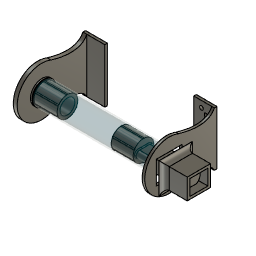
door-window-v3 (Autodesk Fusion 360 design; units mm, degrees)
Autodesk Fusion 360 part; units mm, degrees
note: some values were not read from the file. Chosen so that the rebuilt part matches the saved one: which face or edge a step refers to. Set by a fixed rule: which sketch regions a step uses.
sketch "left holder" plane through (0, 0, 0) normal (1, 0, 0) x (0, 1, 0)
  circle A0 centre (0, 0) radius 8
  circle A1 centre (0, 0) radius 9
  line L0 (0, 0) -> (36, 0) construction
  line L1 (35, 21) -> (37, 21)
  line L2 (37, 21) -> (37, -21)
  line L3 (37, -21) -> (35, -21)
  line L4 (35, -21) -> (35, 21)
  line L5 (35, 21) -> (37, -21) construction
  line L6 (37, 21) -> (35, -21) construction
  circle A2 centre (0, 0) radius 19
  spline S0 degree 5 poles (7.0865, 17.629) (9.067, 17.0403) (12.8106, 16.0316) (17.775, 15.0239) (23.2427, 14.5868) (28.5965, 15.294) (31.8536, 16.8398) (33.6847, 18.6426) (34.6107, 20.1614) (35, 21) knots 0 0 0 0 0 0 0.2 0.4 0.6 0.8 1 1 1 1 1 1
  line L7 (2.4318, 19.0126) -> (11.7413, 16.2454)
  line L8 (34.2297, 19.3403) -> (35.7703, 22.6597)
  spline S1 degree 5 poles (7.0865, -17.629) (9.067, -17.0403) (12.8106, -16.0316) (17.775, -15.0239) (23.2427, -14.5868) (28.5965, -15.294) (31.8536, -16.8398) (33.6847, -18.6426) (34.6107, -20.1614) (35, -21) knots 0 0 0 0 0 0 0.2 0.4 0.6 0.8 1 1 1 1 1 1
  line L9 (2.4318, -19.0126) -> (11.7413, -16.2454)
  line L10 (34.2297, -19.3403) -> (35.7703, -22.6597)
  circle A3 centre (0, 0) radius 3
  point P0 (36, 0)
  dimension "d1" = 16
  dimension "d2" = 18
  dimension "d3" = 36
  dimension "d4" = 2
  dimension "d5" = 42
  dimension "d8" = 38
  dimension "d9" = 6
  constraint coincident A0.centre A1.centre
  constraint concentric A0 A1
  constraint horizontal L0
  constraint horizontal L1
  constraint perpendicular L1 L2
  constraint parallel L1 L3
  constraint parallel L2 L4
  constraint coincident L5 P0
  constraint coincident L6 P0
  constraint coincident P0 L0.end
  constraint concentric A1 A2
  constraint coincident A2 S0.start
  constraint midpoint S0.start L7
  constraint midpoint L1.start L8
  constraint symmetric L0 L1.start L3.end
  constraint symmetric L0 S0.start S1.start
  constraint symmetric L0 L7.start L9.start
  constraint symmetric L0 L7.end L9.end
  constraint symmetric L0 L8.start L10.start
  constraint symmetric L0 L8.end L10.end
  measures "d1" diameter of A0
  measures "d2" diameter of A1
  measures "d3" distance of A0.centre P0
  measures "d4" distance of L2.end L3.end
  measures "d5" distance of L1.end L2.end
  measures "d8" diameter of A2
  measures "d9" diameter of A3
extrude "Extrude1" add sketch "left holder" along normal blind 17 contours L1 L2 L3 L4 makes body 1
extrude "Extrude3" add sketch "left holder" along normal blind 2 contours A0 | A1 | L4 A2 S0 S1 | A2 L7 | A2 L7 L9 | A2 L9 bodies 1
extrude "Extrude4" add sketch "left holder" along normal blind 90 from surface at 5 separate body contours A1 makes body 2
extrude "Extrude5" add sketch "left holder" along normal blind 10 from surface at 3 separate body contours A0 | A3 makes body 3
extrude "Extrude6" add sketch "left holder" against normal blind 4 from surface at 3 contours A3 bodies 3
extrude "Extrude7" add sketch "left holder" along normal blind 3 contours A0 bodies 1
fillet "Fillet1" radius 1 1 edges at (3, -7.4586, -2.8929) on bodies 1
extrude "Extrude8" add 1 faces at (5, 8.6034, -0.8446) along direction (-1, 0, 0) blind 1.2 from surface at 0.5 separate body on bodies 2 makes body 4
combine "Combine1" operation add target body 4 tool bodies 3
move_face "OffsetFaces1" offset 2 1 faces at (-1, -1.1591, 0.5829) on bodies 4
sketch "left inside" plane through (13, 0, 0) normal (1, 0, 0) x (0, 1, 0)
  circle A0 centre (0, 0) radius 8
  circle A1 centre (0, 0) radius 7.75
  circle A2 centre (0, 0) radius 5.75
  circle A3 centre (0, 7.75) radius 0.5227
  circle A4 centre (-6.7117, 3.875) radius 0.5227
  circle A5 centre (-6.7117, -3.875) radius 0.5227
  circle A6 centre (0, -7.75) radius 0.5227
  circle A7 centre (6.7117, -3.875) radius 0.5227
  circle A8 centre (6.7117, 3.875) radius 0.5227
  dimension "d31" = -2
  dimension "d35" = 360
  dimension "d38" = 15.5
  constraint coincident A0.centre A1.centre
  constraint coincident A1 A3.centre
  measures "d38" diameter of A1
extrude "Extrude9" cut sketch "left inside" against normal blind 7 contours A2 bodies 4
extrude "Extrude10" add sketch "left inside" against normal blind 8.5 contours A0 A1 A8 | A0 A8 | A0 A7 | A0 A1 A7 | A0 A1 A3 A8 | A0 A1 A6 A7 | A0 A1 A3 | A0 A3 | A0 A6 | A0 A1 A6 | A0 A1 A3 A4 | A0 A1 A5 A6 | A0 A1 A4 | A0 A4 | A0 A5 | A0 A1 A5 | A0 A1 A4 A5 bodies 4
extrude "Extrude2" add sketch "left holder" along normal blind 3 contours A0 | A1 | L4 A2 S0 S1 | A2 L7 | A2 L7 L9 | A2 L9 bodies 1
move_face "OffsetFaces2" offset -1 1 faces at (3, 6.2924, 0.5465) on bodies 4
move_face "OffsetFaces3" offset 10 1 faces at (13, -3.6191, 6.2685) on bodies 4
copy_body "CopyPasteBodies1" bodies 4 makes body 5
move_body "Move1" bodies 5 to x (-1, 0, 0) y (0, 1, 0) z (0, 0, -1) at (88, 0, 0)
move_face "OffsetFaces4" offset -7 1 faces at (91, 1.2818, 1.0989) on bodies 5
sketch "Sketch3" plane through (84, 0, 0) normal (1, 0, 0) x (0, 1, 0)
  circle A0 centre (0, 0) radius 8
  line L0 (-4, -3) -> (4, -3)
  arc A1 (4, -3) -> (4, 3) centre (4, 0) ccw
  line L1 (4, 3) -> (-4, 3)
  arc A2 (-4, 3) -> (-4, -3) centre (-4, 0) ccw
  line L2 (-4, 0) -> (4, 0) construction
  line L3 (-4, -2.6) -> (4, -2.6)
  arc A3 (4, -2.6) -> (4, 2.6) centre (4, 0) ccw
  line L4 (4, 2.6) -> (-4, 2.6)
  arc A4 (-4, 2.6) -> (-4, -2.6) centre (-4, 0) ccw
  circle A5 centre (0, 0) radius 1.5
  line L5 (0, 1.5) -> (0, -0.9)
  line L6 (-1.2, -0.9) -> (1.2, -0.9)
  dimension "d45" = 4
  dimension "d50" = 3
  dimension "d53" = -0.4
  dimension "d58" = 3
  dimension "d59" = 2.4
  constraint tangent L0 A1
  constraint tangent A1 L1
  constraint parallel L0 L1
  constraint tangent L1 A2
  constraint tangent L0 A2
  constraint horizontal L2
  constraint coincident A0.centre A5.centre
  constraint midpoint L2 A0.centre
  constraint coincident A5 L5.start
  constraint perpendicular L4 L5
  constraint coincident A5 L6.start
  constraint coincident A5 L6.end
  constraint perpendicular L5 L6
  measures "d45" distance of A2.centre A0.centre
  measures "d50" distance of A0.centre L1
  measures "d58" diameter of A5
  measures "d59" distance of L5.start L5.end
extrude "Extrude11" cut 1 faces at (82, -1.5948, -0.4036) along direction (1, 0, 0) blind 9.5 on bodies 5 bodies 5
move_face "OffsetFaces5" offset -2.5 1 faces at (84.7, 8.6034, 0.8446) on bodies 5
extrude "Extrude12" cut sketch "Sketch3" against normal blind 19 contours L0 A1 L1 A2 | L3 A3 L4 A4 | A5 L5 L6 | A5 L5 L6 | A5 L6 bodies 5
extrude "Extrude13" add sketch "Sketch3" against normal blind 19 contours A0 bodies 5
extrude "Extrude14" cut sketch "Sketch3" against normal blind 2 contours A0 bodies 5
extrude "Extrude16" add sketch "Sketch3" along normal blind 12 separate body contours L3 A3 L4 A4 | A5 L5 L6 | A5 L5 L6 | A5 L6 makes body 6
extrude "Extrude17" cut sketch "Sketch3" against normal blind 6.5 from surface at 12 contours A5 L5 L6 | A5 L5 L6 bodies 6
extrude "Extrude18" add sketch "Sketch3" against normal blind 6 from surface at 12 separate body contours A5 L5 L6 | A5 L5 L6 makes body 7
sketch "Sketch4" plane through (96, 0, 0) normal (1, 0, 0) x (0, 1, 0)
  arc A0 (1.2, -0.9) -> (-1.2, -0.9) centre (0, 0) ccw
  line L0 (-1.2, -0.9) -> (1.2, -0.9)
  circle A1 centre (0, 0) radius 1.5
  line L1 (6, 5) -> (-6, 5)
  line L2 (-6, 5) -> (-6, -5)
  line L3 (-6, -5) -> (6, -5)
  line L4 (6, -5) -> (6, 5)
  line L5 (6, 5) -> (-6, -5) construction
  line L6 (-6, 5) -> (6, -5) construction
  arc A2 (-3.3166, 5) -> (-3.3166, -5) centre (0, 0) ccw
  arc A3 (3.3166, -5) -> (3.3166, 5) centre (0, 0) ccw
  dimension "d66" = 3
  dimension "d67" = 12
  dimension "d68" = 10
  constraint coincident A0.centre A1.centre
  constraint horizontal L1
  constraint perpendicular L1 L2
  constraint parallel L1 L3
  constraint parallel L2 L4
  constraint coincident L5 A0.centre
  constraint coincident L6 A0.centre
  constraint tangent L2 A2
  constraint coincident L1 A3.end
  constraint coincident L1 A2.start
  constraint coincident L3 A2.end
  constraint coincident L3 A3.start
  constraint concentric A2 A3
  measures "d66" diameter of A1
  measures "d67" distance of L2.end L3.end
  measures "d68" distance of L1.end L2.end
extrude "Extrude19" add sketch "Sketch4" along normal blind 24 contours A0 L0 A1 | L0 A1 | L1 L4 A3 | L1 L3 A2 A3 | L3 L4 A3 | L1 L2 A2 | L2 L3 A2 bodies 7
extrude "Extrude21" cut sketch "Sketch4" against normal blind 10 from surface at 24 contours L1 L4 A3 | L3 L4 A3 | L1 L2 A2 | L2 L3 A2 bodies 7
move_body "Move2" bodies 6 to x (1, 0, 0) y (0, 1, 0) z (0, 0, 1) at (-1, 0, 0)
sketch "Sketch5" plane through (96, 0, 0) normal (-1, 0, 0) x (0, -1, 0)
  line L0 (-6, 5) -> (-6, -5)
  line L1 (-6, -5) -> (6, -5)
  line L2 (6, -5) -> (6, 5)
  line L3 (6, 5) -> (-6, 5)
  line L4 (1.2, -0.9) -> (-1.2, -0.9)
  arc A0 (1.2, -0.9) -> (-1.2, -0.9) centre (0, 0) ccw
  line L5 (7, -6) -> (-7, -6)
  line L6 (-7, -6) -> (-7, 6)
  line L7 (-7, 6) -> (7, 6)
  line L8 (7, 6) -> (7, -6)
  line L9 (7, -6) -> (-7, 6) construction
  line L10 (-7, -6) -> (7, 6) construction
  line L11 (9, -8) -> (-9, -8)
  line L12 (-9, -8) -> (-9, 8)
  line L13 (-9, 8) -> (9, 8)
  line L14 (9, 8) -> (9, -8)
  dimension "d77" = 14
  dimension "d78" = 12
  dimension "d79" = -2
  constraint horizontal L5
  constraint perpendicular L5 L6
  constraint parallel L5 L7
  constraint parallel L6 L8
  constraint coincident L9 A0.centre
  constraint coincident L10 A0.centre
  constraint coincident A0.centre origin
  measures "d77" distance of L6.end L7.end
  measures "d78" distance of L5.end L6.end
extrude "Extrude22" add sketch "Sketch5" along normal blind 20 from surface at -24 separate body contours L11 L12 L13 L14 makes body 8
extrude "Extrude23" add sketch "left holder" along normal blind 2 from surface at 100 contours A0 | A1 | L1 L2 L3 L4 | L4 A2 S0 S1 | A2 L7 | A2 L7 L9 | A2 L9 bodies 8
extrude "Extrude24" cut 1 faces at (102, -5.6667, 0) along direction (-1, 0, 0) blind 2 on bodies 8 bodies 8
extrude "Extrude25" add 1 faces at (17, 35.6667, 7) along direction (-1, 0, 0) blind 16 from surface at -85 on bodies 1 bodies 1 8
sketch "Sketch6" plane through (0, 0, -21) normal (0, 0, -1) x (1, 0, 0)
  line L0 (86, -37) -> (102, -37)
  line L1 (102, -37) -> (102, -35)
  line L2 (102, -35) -> (100, -35)
  line L3 (100, -35) -> (86, -35)
  line L4 (86, -35) -> (86, -37)
  spline S0 degree 5 poles (100, -25) (99.9495, -25.3953) (99.8279, -26.1864) (99.5842, -27.3747) (99.1279, -28.9626) (98.2314, -30.9562) (97.089, -32.5626) (95.8729, -33.7769) (94.8769, -34.5915) (94.3325, -35) knots 0 0 0 0 0 0 0.2 0.4 0.6 0.8 1 1 1 1 1 1
  line L5 (95.665, -34) -> (93, -36)
  line L6 (94.3325, -35) -> (100, -35)
  line L7 (94.3325, -35) -> (100, -35)
  line L8 (100, -25) -> (100, -35)
  constraint coincident L3 S0.end
  constraint midpoint S0.end L5
  constraint coincident L2.end L3.start
extrude "Extrude26" add sketch "Sketch6" along normal blind 2 separate body contours L3 S0 L6 L7 L8 makes body 9
pattern_linear "R-Pattern1" count 5 spacing 8.75 along (0, 0, 1) of bodies 9 makes body 10 at (97.6571, 31.6501, -13.213) makes body 11 at (97.6571, 31.6501, -4.463) makes body 12 at (97.6571, 31.6501, 4.287) makes body 13 at (97.6571, 31.6501, 13.037)
combine "Combine2" operation add target body 10 tool bodies 13 12 8 11
sketch "Sketch7" plane through (0, 35, 0) normal (0, -1, 0) x (1, 0, 0)
  line L0 (100, -5.5) -> (94.3325, -5.5)
  line L1 (94.3325, -5.5) -> (94.3325, -3.5)
  line L2 (94.3325, -3.5) -> (100, -3.5)
  line L3 (100, -3.5) -> (100, 3.25)
  line L4 (100, 3.25) -> (94.3325, 3.25)
  line L5 (94.3325, 3.25) -> (94.3325, 5.25)
  line L6 (94.3325, 5.25) -> (100, 5.25)
  line L7 (100, 5.25) -> (100, 12)
  line L8 (100, 12) -> (94.3325, 12)
  line L9 (94.3325, 12) -> (94.3325, 14)
  line L10 (94.3325, 14) -> (100, 14)
  line L11 (100, 14) -> (100, 21)
  line L12 (100, 21) -> (86, 21)
  line L13 (86, 21) -> (86, -21)
  line L14 (86, -21) -> (100, -21)
  line L15 (100, -21) -> (100, -14.25)
  line L16 (100, -14.25) -> (94.3325, -14.25)
  line L17 (94.3325, -14.25) -> (94.3325, -12.25)
  line L18 (94.3325, -12.25) -> (100, -12.25)
  line L19 (100, -12.25) -> (100, -5.5)
  line L20 (86, 17.3093) -> (92, 17.3093) construction
  line L21 (89.5567, 21) -> (89.5567, 16)
  circle A0 centre (92, 16) radius 1.5
  dimension "d97" = 6
  dimension "d98" = 5
  dimension "d99" = 3
  constraint coincident L13 L20.start
  constraint perpendicular L13 L20
  constraint coincident L12 L21.start
  constraint perpendicular L20 L21
  measures "d97" distance of L20.start L20.end
  measures "d98" distance of L21.start L21.end
  measures "d99" diameter of A0
extrude "Extrude27" cut sketch "Sketch7" against normal blind 2 contours A0 bodies 10
pattern_linear "R-Pattern2" count 2 spacing 22 along (0, 0, -1) of "Extrude27"
fillet "Fillet2" radius 4 4 edges at (102, 0, 8) (102, -9, 0) (102, 9, 0) (102, 0, -8) on bodies 10
split "Split1" by plane through (102, 0, 0) normal (1, 0, 0) bodies 10 makes body 14 at (110.6667, -3, -8)
move_body "Move3" bodies 14 to x (1, 0, 0) y (0, 1, 0) z (0, 0, 1) at (5, 0, 0)
sketch "Sketch9" plane through (107, 0, 0) normal (-1, 0, 0) x (0, -1, 0)
  line L0 (13, 12) -> (-13, 12)
  line L1 (-13, 12) -> (-13, -12)
  line L2 (-13, -12) -> (13, -12)
  line L3 (13, -12) -> (13, 12)
  line L4 (7, -6) -> (-7, -6)
  line L5 (-7, -6) -> (-7, 6)
  line L6 (-7, 6) -> (7, 6)
  line L7 (7, 6) -> (7, -6)
  line L8 (-7, 6) -> (7, 6)
  line L9 (7, 6) -> (7, -6)
  line L10 (7, -6) -> (-7, -6)
  line L11 (-7, -6) -> (-7, 6)
  line L12 (10, -9) -> (-10, -9)
  line L13 (-10, -9) -> (-10, 9)
  line L14 (-10, 9) -> (10, 9)
  line L15 (10, 9) -> (10, -9)
  line L16 (10, 9) -> (-10, 9)
  line L17 (-10, 9) -> (-10, -9)
  line L18 (-10, -9) -> (10, -9)
  line L19 (10, -9) -> (10, 9)
  line L20 (-9.8, -8.8) -> (9.8, -8.8)
  line L21 (9.8, -8.8) -> (9.8, 8.8)
  line L22 (9.8, 8.8) -> (-9.8, 8.8)
  line L23 (-9.8, 8.8) -> (-9.8, -8.8)
  dimension "d108" = -3
  dimension "d114" = -0.2
  constraint horizontal L8
  constraint vertical L9
  constraint horizontal L10
  constraint vertical L11
  constraint coincident L4.start L7.end
  constraint coincident L5.end L6.start
  constraint horizontal L16
  constraint vertical L17
  constraint horizontal L18
  constraint vertical L19
extrude "Extrude28" add sketch "Sketch9" along normal blind 2 contours L12 L13 L14 L15 L16 L17 L18 L19 | L20 L21 L22 L23 bodies 14
extrude "Extrude29" cut sketch "Sketch9" against normal blind 2 from surface at 7 contours L12 L13 L14 L15 L16 L17 L18 L19 | L20 L21 L22 L23 bodies 10
extrude "Extrude30" cut sketch "Sketch9" along normal blind 2 contours L12 L13 L14 L15 L16 L17 L18 L19 bodies 14
copy_body "CopyPasteBodies2" bodies 5 makes body 15
move_body "Move4" bodies 15 to x (1, 0, 0) y (0, 1, 0) z (0, 0, 1) at (0, 35.6342, 35.0743)
copy_body "CopyPasteBodies3" bodies 6 makes body 16
move_body "Move5" bodies 16 to x (1, 0, 0) y (0, 1, 0) z (0, 0, 1) at (0, 0, 145)
hidden bodies 9 15 16
named bodies: "holder", "tube", "inside-tube", "inside left", "inside left (1)", "motor-holder-right", "motor-holder-right (1)", "inside left (1) (1)"
